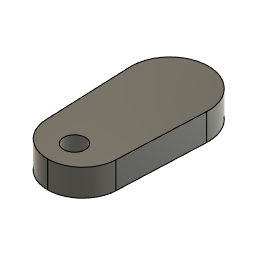
AnetA8RodEnd (Autodesk Fusion 360 design; units mm, degrees)
Autodesk Fusion 360 part; units mm, degrees
sketch "Sketch1" plane through (0, 0, 0) normal (0, 1, 0) x (1, 0, 0)
  line L0 (-0.0152, -15) -> (0.0152, -15)
  line L1 (0.0062, 15) -> (-0.0062, 15)
  line L2 (0, 15) -> (0, -15) construction
  line L3 (-7.1875, 7.5003) -> (-6.5096, -8.7706)
  line L4 (7.1875, 7.5003) -> (6.5096, -8.7706)
  arc A0 (0.0062, 15) -> (-7.1875, 7.5003) centre (0.0062, 7.8) ccw
  arc A1 (7.1875, 7.5003) -> (-0.0062, 15) centre (-0.0062, 7.8) ccw
  arc A2 (-6.5096, -8.7706) -> (-0.0152, -15) centre (-0.0152, -8.5) ccw
  arc A3 (0.0152, -15) -> (6.5096, -8.7706) centre (0.0152, -8.5) ccw
  point P0 (-6.25, -15)
  point P1 (6.25, -15)
  point P2 (-7.5, 15)
  point P3 (7.5, 15)
  dimension "d1" = 12.5
  dimension "d2" = 15
  dimension "d3" = 30
  dimension "d4" = 15
  dimension "d6" = 7.2
  dimension "d7" = 6.5
  constraint horizontal L0
  constraint horizontal L1
  constraint perpendicular L1 L2
  constraint coincident L1 L2.start
  constraint coincident P2 L1
  constraint coincident P2 L3
  constraint tangent L1 A0
  constraint tangent L3 A0
  constraint coincident P3 L1
  constraint coincident P3 L4
  constraint tangent L1 A1
  constraint tangent L4 A1
  constraint equal A0 A1
  constraint coincident L0 L2.end
  constraint coincident P0 L0
  constraint coincident P0 L3
  constraint tangent L0 A2
  constraint tangent L3 A2
  constraint coincident P1 L0
  constraint coincident P1 L4
  constraint tangent L0 A3
  constraint tangent L4 A3
  constraint equal A2 A3
  measures "d1" distance of P0 P1
  measures "d2" distance of P2 P3
  measures "d3" distance of L2.start L2.end
  measures "d4" vertical distance of origin L2.start
  measures "d6" radius of A0
  measures "d7" radius of A2
extrude "Extrude1" add sketch "Sketch1" along normal blind 5
sketch "Sketch2" plane through (0, 5, 0) normal (0, 1, 0) x (-1, 0, 0)
  arc A0 (-7.1875, -7.5003) -> (0, -15) centre (0.0062, -7.8) ccw
  arc A1 (0, -15) -> (7.1875, -7.5003) centre (-0.0062, -7.8) ccw
  line L0 (7.1875, -7.5003) -> (6.5096, 8.7706)
  arc A2 (6.5096, 8.7706) -> (0.0152, 15) centre (0.0152, 8.5) ccw
  line L1 (0.0152, 15) -> (-0.0152, 15)
  arc A3 (-0.0152, 15) -> (-6.5096, 8.7706) centre (-0.0152, 8.5) ccw
  line L2 (-6.5096, 8.7706) -> (-7.1875, -7.5003)
  line L3 (-0.0152, 15) -> (-0.0152, 10) construction
  circle A4 centre (-0.0152, 10) radius 2
  dimension "d10" = 5
  dimension "d11" = 4
  constraint coincident L1.end A3.start
  constraint perpendicular L1 L3
  constraint coincident L3.end A4.centre
  measures "d10" distance of L1.end L3.end
  measures "d11" diameter of A4
extrude "Extrude2" cut sketch "Sketch2" against normal blind 7 contours A4
